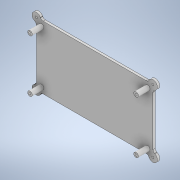
# Autodesk Inventor part: cover_bottom_v3
Saved by Autodesk Inventor 2022 (Build 260153000, 153)
## iProperties
Created: 2022-08-26
Part Number: cover_bottom_v3
Material: Generic
Document SubType Name: Modeling
Designer: suerfu
Density: 1 g/cm^3
Appearance: Default
Author: suerfu
Autodesk Inventor part; units mm, degrees
ref_plane "YZ Plane" through (0, 0, 0) normal (1, 0, 0) x (0, 1, 0)
ref_plane "XZ Plane" through (0, 0, 0) normal (0, 1, 0) x (-1, 0, 0)
ref_plane "XY Plane" through (0, 0, 0) normal (0, 0, 1) x (1, 0, 0)
sketch "Sketch1" plane through (0, 0, 0) normal (0, 0, 1) x (1, 0, 0)
  line L0 (-56.2118, 34.29) -> (63.5, 34.29)
  line L1 (63.5, 34.29) -> (63.5, -34.29)
  line L2 (63.5, -34.29) -> (-63.5, -34.29)
  line L3 (-63.5, -34.29) -> (-63.5, 27.0018)
  line L4 (0, 0) -> (-113.7275, 61.4128) construction
  line L5 (-60.325, 31.115) -> (60.325, 31.115)
  line L6 (60.325, 31.115) -> (60.325, -31.115)
  line L7 (60.325, -31.115) -> (-60.325, -31.115)
  line L8 (-60.325, -31.115) -> (-60.325, 31.115)
  circle A0 centre (-63.5, 34.29) radius 4.7625
  line L9 (-59.0352, 35.9473) -> (-59.1884, 36.3601)
  line L10 (-65.1573, 29.8252) -> (-65.5701, 29.9784)
  arc A1 (-63.5, 27.0018) -> (-65.5701, 29.9784) centre (-66.675, 27.0018) ccw
  arc A2 (-59.1884, 36.3601) -> (-56.2118, 34.29) centre (-56.2118, 37.465) ccw
  line L11 (0, 55.5625) -> (0, -55.5625) construction
  line L12 (-104.775, 0) -> (104.775, 0) construction
  circle A3 centre (63.5, 34.29) radius 4.7625
  line L13 (59.0352, 35.9473) -> (59.1884, 36.3601)
  line L14 (65.1573, 29.8252) -> (65.5701, 29.9784)
  arc A4 (65.5701, 29.9784) -> (63.5, 27.0018) centre (66.675, 27.0018) ccw
  arc A5 (56.2118, 34.29) -> (59.1884, 36.3601) centre (56.2118, 37.465) ccw
  line L15 (104.775, 0) -> (-104.775, 0) construction
  circle A6 centre (-63.5, -34.29) radius 4.7625
  line L16 (-59.0352, -35.9473) -> (-59.1884, -36.3601)
  line L17 (-65.1573, -29.8252) -> (-65.5701, -29.9784)
  arc A7 (-65.5701, -29.9784) -> (-63.5, -27.0018) centre (-66.675, -27.0018) ccw
  arc A8 (-56.2118, -34.29) -> (-59.1884, -36.3601) centre (-56.2118, -37.465) ccw
  circle A9 centre (63.5, -34.29) radius 4.7625
  line L18 (65.1573, -29.8252) -> (65.5701, -29.9784)
  arc A10 (63.5, -27.0018) -> (65.5701, -29.9784) centre (66.675, -27.0018) ccw
  line L19 (59.0352, -35.9473) -> (59.1884, -36.3601)
  arc A11 (59.1884, -36.3601) -> (56.2118, -34.29) centre (56.2118, -37.465) ccw
  line L20 (-30.2895, 0.635) -> (45.0215, 0.635) construction
  line L21 (45.0215, 0.635) -> (45.0215, -27.94) construction
  line L22 (45.0215, -27.94) -> (-30.2895, -27.94) construction
  line L23 (-30.2895, -27.94) -> (-30.2895, 0.635) construction
  line L24 (-47.625, 28.575) -> (47.625, 28.575) construction
  line L25 (47.625, 28.575) -> (47.625, 17.145) construction
  line L26 (47.625, 17.145) -> (-47.625, 17.145) construction
  line L27 (-47.625, 17.145) -> (-47.625, 28.575) construction
  point P0 (-58.42, 34.29)
  point P1 (-63.5, 29.21)
  point P2 (56.2118, 34.29)
  point P3 (-63.5, -27.0018)
  point P4 (-56.2118, -34.29)
  point P5 (56.2118, -34.29)
  point P6 (63.5, -27.0018)
  point P7 (63.5, 27.0018)
  point P8 (-59.9502, -31.115)
  point P9 (-60.325, -30.7402)
  point P10 (59.9502, -31.115)
  point P11 (60.325, -30.7402)
  point P12 (-60.325, 30.7402)
  point P13 (-59.9502, 31.115)
  point P14 (-66.6527, 30.7204)
  point P15 (-66.6527, -30.7204)
  point P16 (66.6527, -30.7204)
  point P17 (66.6527, 30.7204)
  point P18 (-64.4148, 29.6162)
  point P19 (-64.4148, -29.6162)
  point P20 (64.4148, -29.6162)
  point P21 (64.4148, 29.6162)
  dimension "d8" = 63.5
  dimension "d9" = 63.5
  dimension "d10" = 34.29
  dimension "d11" = 34.29
  dimension "d15" = 60.325
  dimension "d16" = 60.325
  dimension "d17" = 62.23
  dimension "d18" = 31.115
  dimension "d19" = 9.525
  dimension "d20" = 5.08
  dimension "d21" = 5.08
  dimension "d22" = 3.175
  dimension "d25" = 48.26
  dimension "d26" = 59.69
  dimension "d27" = 12.7
  dimension "d28" = 107.95
  dimension "d29" = 30.0355
  dimension "d30" = 105.3465
  dimension "d31" = 3.175
  dimension "d32" = 31.75
  constraints: 56 end point, 29 symmetric about line, 24 point on circle, 12 centre point, 8 parallel, 7 point on line, 6 tangent, 5 horizontal, 4 perpendicular, 1 coincident, 1 equal radius, 1 vertical, 9 other
  measures "d8" distance from line of L4.start L3
  measures "d9" distance from line of L1 L4.start
  measures "d10" distance from line of L4.start L2
  measures "d11" distance from line of L0 L4.start
  measures "d15" distance from line of L4.start L8
  measures "d16" distance from line of L4.start L6
  measures "d17" distance between parallel lines of L7 L5
  measures "d18" distance from line of L4.start L5
  measures "d19" diameter of A0
  measures "d20" distance of point (-58.42, 34.29) point (-63.5, 34.29)
  measures "d21" distance of point (-63.5, 34.29) point (-63.5, 29.21)
  measures "d22" radius of A1
  measures "d25" distance between parallel lines of L26 L7
  measures "d26" distance between parallel lines of L24 L7
  measures "d27" distance between parallel lines of L8 L27
  measures "d28" distance between parallel lines of L8 L25
  measures "d29" distance between parallel lines of L8 L23
  measures "d30" distance between parallel lines of L8 L21
  measures "d31" distance between parallel lines of L22 L7
  measures "d32" distance between parallel lines of L20 L7
extrude "Extrusion1" add sketch "Sketch1" along normal blind 2.54
sketch "Sketch2" plane through (0, 0, 2.54) normal (0, 0, 1) x (1, 0, 0)
  circle A0 centre (-63.5, 34.29) radius 2.2451
  circle A1 centre (-63.5, -34.29) radius 1.7045
  circle A2 centre (63.5, 34.29) radius 1.7045
  circle A3 centre (63.5, -34.29) radius 1.5875
  arc A4 (-59.0352, 35.9473) -> (-65.1573, 29.8252) centre (-63.5, 34.29) ccw projected
  arc A5 (-65.1573, -29.8252) -> (-59.0352, -35.9473) centre (-63.5, -34.29) ccw projected
  arc A6 (65.1573, 29.8252) -> (59.0352, 35.9473) centre (63.5, 34.29) ccw projected
  arc A7 (59.0352, -35.9473) -> (65.1573, -29.8252) centre (63.5, -34.29) ccw projected
  point P0 (0, 0)
  point P1 (-66.6527, 30.7204)
  point P2 (-66.6527, -30.7204)
  point P3 (66.6527, 30.7204)
  point P4 (66.6527, -30.7204)
  point P5 (-64.4148, 29.6162)
  point P6 (-64.4148, -29.6162)
  point P7 (64.4148, 29.6162)
  point P8 (64.4148, -29.6162)
  constraints: 4 centre point, 4 coincident, 4 concentric
hole "Hole1" at (-63.5, -34.29, 2.54) at (-63.5, 34.29, 2.54) at (63.5, 34.29, 2.54) at (63.5, -34.29, 2.54) direction (0, 0, -1) diameter 2.2606 end through all start extended yes clearance for "Socket Head Cap Screw" size "#2" standard "Ansi Unified Screw Threads"
sketch "Sketch3" plane through (0, 0, 2.54) normal (0, 0, 1) x (1, 0, 0)
  line L0 (-60.325, 31.115) -> (60.325, 31.115)
  line L1 (60.325, 31.115) -> (60.325, -31.115)
  line L2 (60.325, -31.115) -> (-60.325, -31.115)
  line L3 (-60.325, -31.115) -> (-60.325, 31.115)
  line L4 (0, 44.45) -> (0, -47.625) construction
  line L5 (-112.7125, 0) -> (95.25, 0) construction
  circle A0 centre (-57.785, 28.575) radius 2.54
  line L6 (60.325, 31.115) -> (-60.325, 31.115)
  circle A1 centre (57.785, 28.575) radius 2.54
  circle A2 centre (-57.785, -28.575) radius 2.54
  circle A3 centre (57.785, -28.575) radius 2.54
  point P0 (0, 0)
  dimension "d40" = 120.65
  dimension "d41" = 62.23
  dimension "d42" = 60.325
  dimension "d43" = 31.115
  dimension "d44" = 5.08
  dimension "d45" = 2.54
  dimension "d46" = 2.54
  constraints: 14 end point, 5 symmetric about line, 4 centre point, 2 horizontal, 2 parallel, 1 perpendicular, 1 vertical, 3 other
  measures "d40" distance of L0.start L0.end
  measures "d41" distance of L2.end L0.start
  measures "d42" distance from line of point (0, 0) L3
  measures "d43" distance from line of point (0, 0) L0
  measures "d44" diameter of A0
  measures "d45" distance from line of L3 A0.centre
  measures "d46" distance from line of L0 A0.centre
extrude "Extrusion2" add sketch "Sketch3" along normal blind 12.7 contours A0 | A1 | A2 | A3
sketch "Sketch4" plane through (-57.785, 28.575, 15.24) normal (0, 0, 1) x (1, 0, 0)
  circle A0 centre (115.57, -57.15) radius 1.0839
  circle A1 centre (115.57, 0) radius 0.8218
  circle A2 centre (0, 0) radius 1.3455
  circle A3 centre (0, -57.15) radius 2.7312
  circle A4 centre (0, 0) radius 2.54 projected
  circle A5 centre (115.57, 0) radius 2.54 projected
  circle A6 centre (115.57, -57.15) radius 2.54 projected
  circle A7 centre (0, -57.15) radius 2.54 projected
  point P0 (57.785, -28.575)
  constraints: 4 centre point, 4 coincident, 4 concentric
hole "Hole2" at (-57.785, 28.575, 15.24) at (-57.785, -28.575, 15.24) at (57.785, 28.575, 15.24) at (57.785, -28.575, 15.24) direction (0, 0, -1) diameter 2.2606 end through all start extended yes clearance for "Socket Head Cap Screw" size "#2" standard "Ansi Unified Screw Threads"
equation "\"d9\" = d8"
equation "\"d11\" = d10"
equation "\"d16\" = d15"
equation "\"d18\" = 0.5 * d17"
equation "\"d20\" = d21"
equation "\"d42\" = 0.5 * d40"
equation "\"d43\" = 0.5 * d41"
body "Solid1"
